rod_end_cap (Autodesk Fusion 360 design; units mm, degrees)
part number: 2026-09-03-23-52-10-226
Autodesk Fusion 360 part; units mm, degrees
sketch "End cap profile" plane through (0, 0, 0) normal (0, 1, 0) x (1, 0, 0)
  line L0 (0, 0) -> (21, 0)
  line L1 (21, 0) -> (21, -4)
  line L2 (21, -4) -> (14.7, -4)
  line L3 (14.7, -4) -> (14.7, -25.5)
  line L4 (14.7, -25.5) -> (12.2, -28)
  line L5 (12.2, -28) -> (0, -28)
  line L6 (0, -28) -> (0, 0)
  dimension "d76" = 21
  dimension "d77" = 4
  dimension "d78" = 14.7
  dimension "d79" = 28
  dimension "d80" = 2.5
  dimension "d81" = 2.5
  constraint horizontal L0
  constraint horizontal L2
  constraint horizontal L5
  constraint vertical L1
  constraint vertical L3
  constraint vertical L6
  constraint coincident L0.start L6.end
  measures "d76" horizontal distance of L0.start L0.end
  measures "d77" vertical distance of L0.end L1.end
  measures "d78" horizontal distance of L0.start L2.end
  measures "d79" vertical distance of L0.start L5.end
  measures "d80" horizontal distance of L3.end L4.end
  measures "d81" vertical distance of L3.end L4.end
revolve "End cap revolve" add sketch "End cap profile" angle 360 about axis through (0, 0, 1.75) along (0, 0, 1)
sketch "Crush rib" plane through (0, 0, 0) normal (0, 1, 0) x (1, 0, 0)
  line L0 (13.7, -5) -> (15.2, -5)
  line L1 (15.2, -5) -> (15.2, -11)
  line L2 (15.2, -11) -> (13.7, -26)
  line L3 (13.7, -26) -> (13.7, -5)
  dimension "d83" = 13.7
  dimension "d84" = 5
  dimension "d85" = 15.2
  dimension "d86" = 26
  dimension "d87" = 11
  constraint horizontal L0
  constraint vertical L1
  constraint vertical L3
  measures "d83" horizontal distance of origin L0.start
  measures "d84" vertical distance of origin L0.start
  measures "d85" horizontal distance of origin L0.end
  measures "d86" vertical distance of origin L2.end
  measures "d87" vertical distance of origin L1.end
extrude "Crush rib (1)" add sketch "Crush rib" along normal mid plane 2
pattern_circular "Crush ribs" count 4 over 360 about axis through (0, 0, 1.75) along (0, 0, 1) of "Crush rib (1)"
equation "rodOuterDiameter = 33.4 mm" comment "pipe OD the flange exceeds"
equation "pipeInnerDiameter = 30.0 mm" comment "MEASURED bore, not the spec"
equation "endCapFlangeProud = 4.3 mm" comment "flange beyond the pipe OD"
equation "endCapFlangeThickness = 4.0 mm" comment "flange thickness"
equation "endCapStemLength = 24.0 mm" comment "stem depth into the bore"
equation "endCapStemDiameter = pipeInnerDiameter - 0.6 mm" comment "slip fit"
equation "endCapRibDiameter = pipeInnerDiameter + 0.4 mm" comment "crush fit on ribs"
equation "endCapTipChamfer = 2.5 mm" comment "lead-in at the stem tip"
equation "endCapRibWidth = 2.0 mm" comment "rib width"
equation "endCapRibCount = 4" comment "ribs around the stem"
equation "endCapRibGripLength = 6.0 mm" comment "full-height rib band"
equation "d76 = rodOuterDiameter / 2 + endCapFlangeProud"
equation "d77 = endCapFlangeThickness"
equation "d78 = endCapStemDiameter / 2"
equation "d79 = endCapFlangeThickness + endCapStemLength"
equation "d80 = endCapTipChamfer"
equation "d81 = endCapTipChamfer"
equation "d83 = endCapStemDiameter / 2 - 1 mm"
equation "d84 = endCapFlangeThickness + 1 mm"
equation "d85 = endCapRibDiameter / 2"
equation "d86 = endCapFlangeThickness + endCapStemLength - 2 mm"
equation "d87 = endCapFlangeThickness + 1 mm + endCapRibGripLength"
equation "d88 = endCapRibWidth"
equation "d90 = endCapRibCount"
named bodies: "rod_end_cap"
